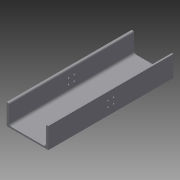
# Autodesk Inventor part: U-Channel Housing 4x2x12
Saved by Autodesk Inventor 2015 (Build 190159000, 159)
## iProperties
Created: 2014-05-17
Part Number: U-Channel Housing 4x2x12
Material: Generic
Document SubType Name: Modeling
Designer: seaha_000
Density: 1 g/cm^3
Appearance: Default
Author: seaha_000
Autodesk Inventor part; units mm, degrees
ref_plane "YZ Plane" through (0, 0, 0) normal (1, 0, 0) x (0, 1, 0)
ref_plane "XZ Plane" through (0, 0, 0) normal (0, 1, 0) x (-1, 0, 0)
ref_plane "XY Plane" through (0, 0, 0) normal (0, 0, 1) x (1, 0, 0)
sketch "Sketch1" plane through (0, 0, 0) normal (0, 0, 1) x (1, 0, 0)
  line L0 (0, 0) -> (50.8, 0)
  line L1 (50.8, 0) -> (50.8, 50.8)
  line L2 (50.8, 50.8) -> (48.133, 50.8)
  line L3 (44.958, 47.625) -> (44.958, 10.16)
  line L4 (0, 0) -> (-50.8, 0)
  line L5 (-50.8, 0) -> (-50.8, 50.8)
  line L6 (-50.8, 50.8) -> (-48.133, 50.8)
  line L7 (-44.958, 47.625) -> (-44.958, 10.16)
  line L8 (-38.608, 3.81) -> (38.608, 3.81)
  arc A0 (-44.958, 10.16) -> (-38.608, 3.81) centre (-38.608, 10.16) ccw
  arc A1 (38.608, 3.81) -> (44.958, 10.16) centre (38.608, 10.16) ccw
  arc A2 (-44.958, 47.625) -> (-48.133, 50.8) centre (-48.133, 47.625) ccw
  arc A3 (48.133, 50.8) -> (44.958, 47.625) centre (48.133, 47.625) ccw
  point P0 (44.958, 50.8)
  point P1 (44.958, 3.81)
  point P2 (49.4665, 50.8)
  point P3 (-44.958, 50.8)
  point P4 (-44.958, 3.81)
  dimension "d0" = 50.8
  dimension "d1" = 50.8
  dimension "d2" = 5.842
  dimension "d3" = 46.99
  dimension "d4" = 50.8
  dimension "d5" = 5.842
  dimension "d6" = 46.99
  dimension "d7" = 50.8
  dimension "d8" = 6.35
  dimension "d9" = 6.35
  dimension "d12" = 3.175
  dimension "d13" = 3.175
  constraints: 18 end point, 8 point on circle, 8 point on line, 8 tangent, 4 centre point, 4 perpendicular, 2 horizontal, 2 vertical, 1 midpoint
  measures "d0" distance of L0.start L0.end
  measures "d1" distance of L0.end L1.end
  measures "d2" distance of L1.end point (44.958, 50.8)
  measures "d3" distance of point (44.958, 50.8) point (44.958, 3.81)
  measures "d4" distance of L0.start L4.end
  measures "d5" distance of L5.end point (-44.958, 50.8)
  measures "d6" distance of point (-44.958, 50.8) point (-44.958, 3.81)
  measures "d7" distance of L4.end L5.end
  measures "d8" radius of A0
  measures "d9" radius of A1
  measures "d12" radius of A2
  measures "d13" radius of A3
extrude "Extrusion1" add sketch "Sketch1" along normal mid plane 304.8
sketch "Sketch3" plane through (50.8, 0, 152.4) normal (1, 0, 0) x (0, 0, -1)
  line L0 (304.8, 50.8) -> (0, 50.8) projected
  line L1 (0, 0) -> (0, 50.8) projected
  line L2 (304.8, 50.8) -> (304.8, 0) projected
  line L3 (0, 25.4) -> (304.8, 25.4) construction
  line L4 (152.4, 50.8) -> (152.4, 0) construction
  circle A0 centre (152.4, 25.4) radius 9.779 construction
  circle A1 centre (159.3148, 32.3148) radius 1.8288
  circle A2 centre (159.3148, 18.4852) radius 1.8288
  circle A3 centre (145.4852, 18.4852) radius 1.8288
  circle A4 centre (145.4852, 32.3148) radius 1.8288
  line L5 (145.4852, 18.4852) -> (159.3148, 18.4852) construction
  line L6 (159.3148, 18.4852) -> (159.3148, 32.3148) construction
  line L7 (159.3148, 32.3148) -> (145.4852, 32.3148) construction
  line L8 (145.4852, 32.3148) -> (145.4852, 18.4852) construction
  line L9 (145.4852, 18.4852) -> (159.3148, 32.3148) construction
  line L10 (159.3148, 18.4852) -> (145.4852, 32.3148) construction
  dimension "d22" = 19.558
  dimension "d23" = 3.6576
  dimension "d24" = 3.6576
  dimension "d25" = 3.6576
  dimension "d26" = 3.6576
  constraints: 16 end point, 6 midpoint, 5 centre point, 4 point on circle, 3 perpendicular, 1 horizontal
  measures "d22" diameter of A0
  measures "d23" diameter of A4
  measures "d24" diameter of A1
  measures "d25" diameter of A3
  measures "d26" diameter of A2
hole "Hole2" at (50.8, 32.3148, 6.9148) at (50.8, 32.3148, -6.9148) at (50.8, 18.4852, -6.9148) at (50.8, 18.4852, 6.9148) direction (-1, 0, 0) diameter 3.81 end through all clearance for "Flat Head Machine Screw (82)" size "#6" standard "Ansi Unified Screw Threads"
equation "\"d4\" = d0"
equation "\"d5\" = d2"
equation "\"d6\" = d3"
equation "\"d7\" = d1"
equation "\"d9\" = d8"
equation "\"d13\" = d12"
equation "\"d24\" = d23"
equation "\"d25\" = d23"
equation "\"d26\" = d23"
body "Solid1"
